Autodesk Fusion 360 part; units mm, degrees
(part 4 of 5)
equation "d84 = FootHeight"
equation "d86 = ( BaseX + LeftRun + FaucetGap ) + ( ( ( RightRun - ModuleGap ) / 2 ) - Wall - 12 mm )"
equation "d87 = ( BaseY ) + ( ( Depth ) - Wall - 12 mm )"
equation "d90 = PanHeight - DeckThick"
equation "d94 = ( BaseX + LeftRun + FaucetGap ) + ( 3 mm )"
equation "d95 = ( BaseY ) + ( 0 mm )"
equation "d96 = RunnerWidth"
equation "d97 = ( Depth ) - 9 mm"
equation "d98 = FootHeight"
equation "d102 = ( BaseX + LeftRun + FaucetGap ) + ( ( ( RightRun - ModuleGap ) / 2 ) - 3 mm - RunnerWidth )"
equation "d103 = ( BaseY ) + ( 0 mm )"
equation "d104 = RunnerWidth"
equation "d105 = ( Depth ) - 9 mm"
equation "d106 = FootHeight"
equation "d108 = TouchChamfer"
equation "d109 = ( FootHeight ) + PanHeight - DeckThick"
equation "d111 = ( BaseX + LeftRun + FaucetGap ) + ( Wall + DeckClearance )"
equation "d112 = ( BaseY ) + ( Wall + DeckClearance )"
equation "d113 = ( ( RightRun - ModuleGap ) / 2 ) - 2 * ( Wall + DeckClearance )"
equation "d114 = ( Depth ) - 2 * ( Wall + DeckClearance )"
equation "d115 = DeckThick"
equation "d117 = ( FootHeight ) + PanHeight - DeckThick"
equation "d119 = ( BaseX + LeftRun + FaucetGap ) + ( ( ( ( ( RightRun - ModuleGap ) / 2 ) - ( 10 * SlotPitch + SlotWidth ) ) / 2 ) + ( 0 * SlotPitch ) )"
equation "d120 = ( BaseY ) + ( Wall + DeckClearance + RimBorder )"
equation "d121 = SlotWidth"
equation "d122 = ( Depth ) - 2 * ( Wall + DeckClearance + RimBorder )"
equation "d123 = DeckThick"
equation "d125 = ( FootHeight ) + PanHeight - DeckThick"
equation "d127 = ( BaseX + LeftRun + FaucetGap ) + ( ( ( ( ( RightRun - ModuleGap ) / 2 ) - ( 10 * SlotPitch + SlotWidth ) ) / 2 ) + ( 1 * SlotPitch ) )"
equation "d128 = ( BaseY ) + ( Wall + DeckClearance + RimBorder )"
equation "d129 = SlotWidth"
equation "d130 = ( Depth ) - 2 * ( Wall + DeckClearance + RimBorder )"
equation "d131 = DeckThick"
equation "d133 = ( FootHeight ) + PanHeight - DeckThick"
equation "d135 = ( BaseX + LeftRun + FaucetGap ) + ( ( ( ( ( RightRun - ModuleGap ) / 2 ) - ( 10 * SlotPitch + SlotWidth ) ) / 2 ) + ( 2 * SlotPitch ) )"
equation "d136 = ( BaseY ) + ( Wall + DeckClearance + RimBorder )"
equation "d137 = SlotWidth"
equation "d138 = ( Depth ) - 2 * ( Wall + DeckClearance + RimBorder )"
equation "d139 = DeckThick"
equation "d141 = ( FootHeight ) + PanHeight - DeckThick"
equation "d143 = ( BaseX + LeftRun + FaucetGap ) + ( ( ( ( ( RightRun - ModuleGap ) / 2 ) - ( 10 * SlotPitch + SlotWidth ) ) / 2 ) + ( 3 * SlotPitch ) )"
equation "d144 = ( BaseY ) + ( Wall + DeckClearance + RimBorder )"
equation "d145 = SlotWidth"
equation "d146 = ( Depth ) - 2 * ( Wall + DeckClearance + RimBorder )"
equation "d147 = DeckThick"
equation "d149 = ( FootHeight ) + PanHeight - DeckThick"
equation "d151 = ( BaseX + LeftRun + FaucetGap ) + ( ( ( ( ( RightRun - ModuleGap ) / 2 ) - ( 10 * SlotPitch + SlotWidth ) ) / 2 ) + ( 4 * SlotPitch ) )"
equation "d152 = ( BaseY ) + ( Wall + DeckClearance + RimBorder )"
equation "d153 = SlotWidth"
equation "d154 = ( Depth ) - 2 * ( Wall + DeckClearance + RimBorder )"
equation "d155 = DeckThick"
equation "d157 = ( FootHeight ) + PanHeight - DeckThick"
equation "d159 = ( BaseX + LeftRun + FaucetGap ) + ( ( ( ( ( RightRun - ModuleGap ) / 2 ) - ( 10 * SlotPitch + SlotWidth ) ) / 2 ) + ( 5 * SlotPitch ) )"
equation "d160 = ( BaseY ) + ( Wall + DeckClearance + RimBorder )"
equation "d161 = SlotWidth"
equation "d162 = ( Depth ) - 2 * ( Wall + DeckClearance + RimBorder )"
equation "d163 = DeckThick"
equation "d165 = ( FootHeight ) + PanHeight - DeckThick"
equation "d167 = ( BaseX + LeftRun + FaucetGap ) + ( ( ( ( ( RightRun - ModuleGap ) / 2 ) - ( 10 * SlotPitch + SlotWidth ) ) / 2 ) + ( 6 * SlotPitch ) )"
equation "d168 = ( BaseY ) + ( Wall + DeckClearance + RimBorder )"
equation "d169 = SlotWidth"
equation "d170 = ( Depth ) - 2 * ( Wall + DeckClearance + RimBorder )"
equation "d171 = DeckThick"
equation "d173 = ( FootHeight ) + PanHeight - DeckThick"
equation "d175 = ( BaseX + LeftRun + FaucetGap ) + ( ( ( ( ( RightRun - ModuleGap ) / 2 ) - ( 10 * SlotPitch + SlotWidth ) ) / 2 ) + ( 7 * SlotPitch ) )"
equation "d176 = ( BaseY ) + ( Wall + DeckClearance + RimBorder )"
equation "d177 = SlotWidth"
equation "d178 = ( Depth ) - 2 * ( Wall + DeckClearance + RimBorder )"
equation "d179 = DeckThick"
equation "d181 = ( FootHeight ) + PanHeight - DeckThick"
equation "d183 = ( BaseX + LeftRun + FaucetGap ) + ( ( ( ( ( RightRun - ModuleGap ) / 2 ) - ( 10 * SlotPitch + SlotWidth ) ) / 2 ) + ( 8 * SlotPitch ) )"
equation "d184 = ( BaseY ) + ( Wall + DeckClearance + RimBorder )"
equation "d185 = SlotWidth"
equation "d186 = ( Depth ) - 2 * ( Wall + DeckClearance + RimBorder )"
equation "d187 = DeckThick"
equation "d189 = ( FootHeight ) + PanHeight - DeckThick"
equation "d191 = ( BaseX + LeftRun + FaucetGap ) + ( ( ( ( ( RightRun - ModuleGap ) / 2 ) - ( 10 * SlotPitch + SlotWidth ) ) / 2 ) + ( 9 * SlotPitch ) )"
equation "d192 = ( BaseY ) + ( Wall + DeckClearance + RimBorder )"
equation "d193 = SlotWidth"
equation "d194 = ( Depth ) - 2 * ( Wall + DeckClearance + RimBorder )"
equation "d195 = DeckThick"
equation "d197 = ( FootHeight ) + PanHeight - DeckThick"
equation "d199 = ( BaseX + LeftRun + FaucetGap ) + ( ( ( ( ( RightRun - ModuleGap ) / 2 ) - ( 10 * SlotPitch + SlotWidth ) ) / 2 ) + ( 10 * SlotPitch ) )"
equation "d200 = ( BaseY ) + ( Wall + DeckClearance + RimBorder )"
equation "d201 = SlotWidth"
equation "d202 = ( Depth ) - 2 * ( Wall + DeckClearance + RimBorder )"
equation "d203 = DeckThick"
equation "d205 = ( FootHeight ) + PanHeight - DeckThick"
equation "d207 = ( BaseX + LeftRun + FaucetGap ) + ( ( ( RightRun - ModuleGap ) / 2 ) / 2 - 8 mm )"
equation "d208 = ( BaseY ) + ( ( Depth ) - Wall - DeckClearance - 4 mm )"
equation "d211 = DeckThick"
equation "d213 = TouchChamfer"
equation "d214 = FootHeight"
equation "d216 = ( BaseX ) + ( 0 mm )"
equation "d217 = ( BaseY ) + ( 0 mm )"
equation "d218 = TowerWidth"
equation "d219 = Depth"
equation "d220 = PanHeight"
equation "d224 = ( BaseX ) + ( Wall )"
equation "d226 = -( -( ( FootHeight ) + FloorMin + ( ( Depth ) - ( Wall ) ) * tan(DrainSlope) ) )"
equation "d227 = ( ( BaseY ) + ( Wall ) )"
equation "d228 = -( -( ( FootHeight ) + FloorMin + ( ( Depth ) - ( Depth ) ) * tan(DrainSlope) ) )"
equation "d229 = ( ( BaseY ) + ( Depth ) )"
equation "d230 = -( -( FootHeight + PanHeight + 1 mm ) )"
equation "d231 = ( TowerWidth ) - 2 * Wall"
equation "d233 = FootHeight"
equation "d235 = ( BaseX ) + ( Wall )"
equation "d236 = ( BaseY ) + ( Wall )"
equation "d239 = PanHeight - DeckThick"
equation "d241 = FootHeight"
equation "d243 = ( BaseX ) + ( Wall )"
equation "d244 = ( BaseY ) + ( ( Depth ) - Wall - 12 mm )"
equation "d247 = PanHeight - DeckThick"
equation "d249 = FootHeight"
equation "d251 = ( BaseX ) + ( ( TowerWidth ) - Wall - 12 mm )"
equation "d252 = ( BaseY ) + ( Wall )"
equation "d255 = PanHeight - DeckThick"
equation "d257 = FootHeight"
equation "d259 = ( BaseX ) + ( ( TowerWidth ) - Wall - 12 mm )"
equation "d260 = ( BaseY ) + ( ( Depth ) - Wall - 12 mm )"
equation "d263 = PanHeight - DeckThick"
equation "d267 = ( BaseX ) + ( 3 mm )"
equation "d268 = ( BaseY ) + ( 0 mm )"
equation "d269 = RunnerWidth"
equation "d270 = ( Depth ) - 9 mm"
equation "d271 = FootHeight"
equation "d275 = ( BaseX ) + ( ( TowerWidth ) - 3 mm - RunnerWidth )"
equation "d276 = ( BaseY ) + ( 0 mm )"
equation "d277 = RunnerWidth"
equation "d278 = ( Depth ) - 9 mm"
equation "d279 = FootHeight"
equation "d281 = TouchChamfer"
equation "d282 = ( FootHeight ) + PanHeight - DeckThick"
equation "d284 = ( BaseX ) + ( Wall + DeckClearance )"
equation "d285 = ( BaseY ) + ( Wall + DeckClearance )"
equation "d286 = ( TowerWidth ) - 2 * ( Wall + DeckClearance )"
equation "d287 = ( Depth ) - 2 * ( Wall + DeckClearance )"
equation "d288 = DeckThick"
equation "d290 = ( FootHeight ) + PanHeight - DeckThick"
equation "d292 = ( BaseX ) + ( ( ( ( TowerWidth ) - ( 14 * SlotPitch + SlotWidth ) ) / 2 ) + ( 0 * SlotPitch ) )"
equation "d293 = ( BaseY ) + ( Wall + DeckClearance + RimBorder )"
equation "d294 = SlotWidth"
equation "d295 = ( Depth ) - 2 * ( Wall + DeckClearance + RimBorder )"
equation "d296 = DeckThick"
equation "d298 = ( FootHeight ) + PanHeight - DeckThick"
equation "d300 = ( BaseX ) + ( ( ( ( TowerWidth ) - ( 14 * SlotPitch + SlotWidth ) ) / 2 ) + ( 1 * SlotPitch ) )"
equation "d301 = ( BaseY ) + ( Wall + DeckClearance + RimBorder )"
equation "d302 = SlotWidth"
equation "d303 = ( Depth ) - 2 * ( Wall + DeckClearance + RimBorder )"
equation "d304 = DeckThick"
equation "d306 = ( FootHeight ) + PanHeight - DeckThick"
equation "d308 = ( BaseX ) + ( ( ( ( TowerWidth ) - ( 14 * SlotPitch + SlotWidth ) ) / 2 ) + ( 2 * SlotPitch ) )"
equation "d309 = ( BaseY ) + ( Wall + DeckClearance + RimBorder )"
equation "d310 = SlotWidth"
equation "d311 = ( Depth ) - 2 * ( Wall + DeckClearance + RimBorder )"
equation "d312 = DeckThick"
equation "d314 = ( FootHeight ) + PanHeight - DeckThick"
equation "d316 = ( BaseX ) + ( ( ( ( TowerWidth ) - ( 14 * SlotPitch + SlotWidth ) ) / 2 ) + ( 3 * SlotPitch ) )"
equation "d317 = ( BaseY ) + ( Wall + DeckClearance + RimBorder )"
equation "d318 = SlotWidth"
equation "d319 = ( Depth ) - 2 * ( Wall + DeckClearance + RimBorder )"
equation "d320 = DeckThick"
equation "d322 = ( FootHeight ) + PanHeight - DeckThick"
equation "d324 = ( BaseX ) + ( ( ( ( TowerWidth ) - ( 14 * SlotPitch + SlotWidth ) ) / 2 ) + ( 4 * SlotPitch ) )"
equation "d325 = ( BaseY ) + ( Wall + DeckClearance + RimBorder )"
equation "d326 = SlotWidth"
equation "d327 = ( Depth ) - 2 * ( Wall + DeckClearance + RimBorder )"
equation "d328 = DeckThick"
equation "d330 = ( FootHeight ) + PanHeight - DeckThick"
equation "d332 = ( BaseX ) + ( ( ( ( TowerWidth ) - ( 14 * SlotPitch + SlotWidth ) ) / 2 ) + ( 5 * SlotPitch ) )"
equation "d333 = ( BaseY ) + ( Wall + DeckClearance + RimBorder )"
equation "d334 = SlotWidth"
equation "d335 = ( Depth ) - 2 * ( Wall + DeckClearance + RimBorder )"
equation "d336 = DeckThick"
equation "d338 = ( FootHeight ) + PanHeight - DeckThick"
equation "d340 = ( BaseX ) + ( ( ( ( TowerWidth ) - ( 14 * SlotPitch + SlotWidth ) ) / 2 ) + ( 6 * SlotPitch ) )"
equation "d341 = ( BaseY ) + ( Wall + DeckClearance + RimBorder )"
equation "d342 = SlotWidth"
equation "d343 = ( Depth ) - 2 * ( Wall + DeckClearance + RimBorder )"
equation "d344 = DeckThick"
equation "d346 = ( FootHeight ) + PanHeight - DeckThick"
equation "d348 = ( BaseX ) + ( ( ( ( TowerWidth ) - ( 14 * SlotPitch + SlotWidth ) ) / 2 ) + ( 7 * SlotPitch ) )"
equation "d349 = ( BaseY ) + ( Wall + DeckClearance + RimBorder )"
equation "d350 = SlotWidth"
equation "d351 = ( Depth ) - 2 * ( Wall + DeckClearance + RimBorder )"
equation "d352 = DeckThick"
equation "d354 = ( FootHeight ) + PanHeight - DeckThick"
equation "d356 = ( BaseX ) + ( ( ( ( TowerWidth ) - ( 14 * SlotPitch + SlotWidth ) ) / 2 ) + ( 8 * SlotPitch ) )"
equation "d357 = ( BaseY ) + ( Wall + DeckClearance + RimBorder )"
equation "d358 = SlotWidth"
equation "d359 = ( Depth ) - 2 * ( Wall + DeckClearance + RimBorder )"
equation "d360 = DeckThick"
equation "d362 = ( FootHeight ) + PanHeight - DeckThick"
equation "d364 = ( BaseX ) + ( ( ( ( TowerWidth ) - ( 14 * SlotPitch + SlotWidth ) ) / 2 ) + ( 9 * SlotPitch ) )"
equation "d365 = ( BaseY ) + ( Wall + DeckClearance + RimBorder )"
equation "d366 = SlotWidth"
equation "d367 = ( Depth ) - 2 * ( Wall + DeckClearance + RimBorder )"
equation "d368 = DeckThick"
equation "d370 = ( FootHeight ) + PanHeight - DeckThick"
equation "d372 = ( BaseX ) + ( ( ( ( TowerWidth ) - ( 14 * SlotPitch + SlotWidth ) ) / 2 ) + ( 10 * SlotPitch ) )"
equation "d373 = ( BaseY ) + ( Wall + DeckClearance + RimBorder )"
equation "d374 = SlotWidth"
equation "d375 = ( Depth ) - 2 * ( Wall + DeckClearance + RimBorder )"
equation "d376 = DeckThick"
equation "d378 = ( FootHeight ) + PanHeight - DeckThick"
equation "d380 = ( BaseX ) + ( ( ( ( TowerWidth ) - ( 14 * SlotPitch + SlotWidth ) ) / 2 ) + ( 11 * SlotPitch ) )"
equation "d381 = ( BaseY ) + ( Wall + DeckClearance + RimBorder )"
equation "d382 = SlotWidth"
equation "d383 = ( Depth ) - 2 * ( Wall + DeckClearance + RimBorder )"
equation "d384 = DeckThick"
equation "d386 = ( FootHeight ) + PanHeight - DeckThick"
equation "d388 = ( BaseX ) + ( ( ( ( TowerWidth ) - ( 14 * SlotPitch + SlotWidth ) ) / 2 ) + ( 12 * SlotPitch ) )"
equation "d389 = ( BaseY ) + ( Wall + DeckClearance + RimBorder )"
equation "d390 = SlotWidth"
equation "d391 = ( Depth ) - 2 * ( Wall + DeckClearance + RimBorder )"
equation "d392 = DeckThick"
equation "d394 = ( FootHeight ) + PanHeight - DeckThick"
equation "d396 = ( BaseX ) + ( ( ( ( TowerWidth ) - ( 14 * SlotPitch + SlotWidth ) ) / 2 ) + ( 13 * SlotPitch ) )"
equation "d397 = ( BaseY ) + ( Wall + DeckClearance + RimBorder )"
equation "d398 = SlotWidth"
equation "d399 = ( Depth ) - 2 * ( Wall + DeckClearance + RimBorder )"
equation "d400 = DeckThick"
equation "d402 = ( FootHeight ) + PanHeight - DeckThick"
equation "d404 = ( BaseX ) + ( ( ( ( TowerWidth ) - ( 14 * SlotPitch + SlotWidth ) ) / 2 ) + ( 14 * SlotPitch ) )"
equation "d405 = ( BaseY ) + ( Wall + DeckClearance + RimBorder )"
equation "d406 = SlotWidth"
equation "d407 = ( Depth ) - 2 * ( Wall + DeckClearance + RimBorder )"
equation "d408 = DeckThick"
equation "d410 = ( FootHeight ) + PanHeight - DeckThick"
equation "d412 = ( BaseX ) + ( ( TowerWidth ) / 2 - 8 mm )"
equation "d413 = ( BaseY ) + ( ( Depth ) - Wall - DeckClearance - 4 mm )"
equation "d416 = DeckThick"
equation "d418 = TouchChamfer"
equation "d419 = FootHeight"
equation "d421 = ( BaseX + TowerWidth + ModuleGap ) + ( 0 mm )"
equation "d422 = ( BaseY ) + ( 0 mm )"
equation "d423 = LeftRun - TowerWidth - ModuleGap"
equation "d424 = Depth"
equation "d425 = PanHeight"
equation "d429 = ( BaseX + TowerWidth + ModuleGap ) + ( Wall )"
equation "d431 = -( -( ( FootHeight ) + FloorMin + ( ( Depth ) - ( Wall ) ) * tan(DrainSlope) ) )"
equation "d432 = ( ( BaseY ) + ( Wall ) )"
equation "d433 = -( -( ( FootHeight ) + FloorMin + ( ( Depth ) - ( Depth ) ) * tan(DrainSlope) ) )"
equation "d434 = ( ( BaseY ) + ( Depth ) )"
equation "d435 = -( -( FootHeight + PanHeight + 1 mm ) )"
equation "d436 = ( LeftRun - TowerWidth - ModuleGap ) - 2 * Wall"
equation "d438 = FootHeight"
equation "d440 = ( BaseX + TowerWidth + ModuleGap ) + ( Wall )"
equation "d441 = ( BaseY ) + ( Wall )"
equation "d444 = PanHeight - DeckThick"
equation "d446 = FootHeight"
equation "d448 = ( BaseX + TowerWidth + ModuleGap ) + ( Wall )"
equation "d449 = ( BaseY ) + ( ( Depth ) - Wall - 12 mm )"
equation "d452 = PanHeight - DeckThick"
equation "d454 = FootHeight"
equation "d456 = ( BaseX + TowerWidth + ModuleGap ) + ( ( LeftRun - TowerWidth - ModuleGap ) - Wall - 12 mm )"
equation "d457 = ( BaseY ) + ( Wall )"
equation "d460 = PanHeight - DeckThick"
equation "d462 = FootHeight"
equation "d464 = ( BaseX + TowerWidth + ModuleGap ) + ( ( LeftRun - TowerWidth - ModuleGap ) - Wall - 12 mm )"
equation "d465 = ( BaseY ) + ( ( Depth ) - Wall - 12 mm )"
equation "d468 = PanHeight - DeckThick"
equation "d472 = ( BaseX + TowerWidth + ModuleGap ) + ( 3 mm )"
equation "d473 = ( BaseY ) + ( 0 mm )"
equation "d474 = RunnerWidth"
equation "d475 = ( Depth ) - 9 mm"
equation "d476 = FootHeight"
equation "d480 = ( BaseX + TowerWidth + ModuleGap ) + ( ( LeftRun - TowerWidth - ModuleGap ) - 3 mm - RunnerWidth )"
equation "d481 = ( BaseY ) + ( 0 mm )"
equation "d482 = RunnerWidth"
equation "d483 = ( Depth ) - 9 mm"
equation "d484 = FootHeight"
equation "d486 = TouchChamfer"
equation "d487 = ( FootHeight ) + PanHeight - DeckThick"
equation "d489 = ( BaseX + TowerWidth + ModuleGap ) + ( Wall + DeckClearance )"
equation "d490 = ( BaseY ) + ( Wall + DeckClearance )"
equation "d491 = ( LeftRun - TowerWidth - ModuleGap ) - 2 * ( Wall + DeckClearance )"
equation "d492 = ( Depth ) - 2 * ( Wall + DeckClearance )"
equation "d493 = DeckThick"
equation "d495 = ( FootHeight ) + PanHeight - DeckThick"
equation "d497 = ( BaseX + TowerWidth + ModuleGap ) + ( ( ( ( LeftRun - TowerWidth - ModuleGap ) - ( 16 * SlotPitch + SlotWidth ) ) / 2 ) + ( 0 * SlotPitch ) )"
equation "d498 = ( BaseY ) + ( Wall + DeckClearance + RimBorder )"
equation "d499 = SlotWidth"
equation "d500 = ( Depth ) - 2 * ( Wall + DeckClearance + RimBorder )"
equation "d501 = DeckThick"
equation "d503 = ( FootHeight ) + PanHeight - DeckThick"
equation "d505 = ( BaseX + TowerWidth + ModuleGap ) + ( ( ( ( LeftRun - TowerWidth - ModuleGap ) - ( 16 * SlotPitch + SlotWidth ) ) / 2 ) + ( 1 * SlotPitch ) )"
equation "d506 = ( BaseY ) + ( Wall + DeckClearance + RimBorder )"
equation "d507 = SlotWidth"
equation "d508 = ( Depth ) - 2 * ( Wall + DeckClearance + RimBorder )"
equation "d509 = DeckThick"
equation "d511 = ( FootHeight ) + PanHeight - DeckThick"
equation "d513 = ( BaseX + TowerWidth + ModuleGap ) + ( ( ( ( LeftRun - TowerWidth - ModuleGap ) - ( 16 * SlotPitch + SlotWidth ) ) / 2 ) + ( 2 * SlotPitch ) )"
equation "d514 = ( BaseY ) + ( Wall + DeckClearance + RimBorder )"
equation "d515 = SlotWidth"
equation "d516 = ( Depth ) - 2 * ( Wall + DeckClearance + RimBorder )"
equation "d517 = DeckThick"
equation "d519 = ( FootHeight ) + PanHeight - DeckThick"
equation "d521 = ( BaseX + TowerWidth + ModuleGap ) + ( ( ( ( LeftRun - TowerWidth - ModuleGap ) - ( 16 * SlotPitch + SlotWidth ) ) / 2 ) + ( 3 * SlotPitch ) )"
equation "d522 = ( BaseY ) + ( Wall + DeckClearance + RimBorder )"
equation "d523 = SlotWidth"
equation "d524 = ( Depth ) - 2 * ( Wall + DeckClearance + RimBorder )"
equation "d525 = DeckThick"
equation "d527 = ( FootHeight ) + PanHeight - DeckThick"
equation "d529 = ( BaseX + TowerWidth + ModuleGap ) + ( ( ( ( LeftRun - TowerWidth - ModuleGap ) - ( 16 * SlotPitch + SlotWidth ) ) / 2 ) + ( 4 * SlotPitch ) )"
equation "d530 = ( BaseY ) + ( Wall + DeckClearance + RimBorder )"
equation "d531 = SlotWidth"
equation "d532 = ( Depth ) - 2 * ( Wall + DeckClearance + RimBorder )"
equation "d533 = DeckThick"
equation "d535 = ( FootHeight ) + PanHeight - DeckThick"
equation "d537 = ( BaseX + TowerWidth + ModuleGap ) + ( ( ( ( LeftRun - TowerWidth - ModuleGap ) - ( 16 * SlotPitch + SlotWidth ) ) / 2 ) + ( 5 * SlotPitch ) )"
equation "d538 = ( BaseY ) + ( Wall + DeckClearance + RimBorder )"
equation "d539 = SlotWidth"
equation "d540 = ( Depth ) - 2 * ( Wall + DeckClearance + RimBorder )"
equation "d541 = DeckThick"
equation "d543 = ( FootHeight ) + PanHeight - DeckThick"
equation "d545 = ( BaseX + TowerWidth + ModuleGap ) + ( ( ( ( LeftRun - TowerWidth - ModuleGap ) - ( 16 * SlotPitch + SlotWidth ) ) / 2 ) + ( 6 * SlotPitch ) )"
equation "d546 = ( BaseY ) + ( Wall + DeckClearance + RimBorder )"
equation "d547 = SlotWidth"
equation "d548 = ( Depth ) - 2 * ( Wall + DeckClearance + RimBorder )"
equation "d549 = DeckThick"
equation "d551 = ( FootHeight ) + PanHeight - DeckThick"
equation "d553 = ( BaseX + TowerWidth + ModuleGap ) + ( ( ( ( LeftRun - TowerWidth - ModuleGap ) - ( 16 * SlotPitch + SlotWidth ) ) / 2 ) + ( 7 * SlotPitch ) )"
equation "d554 = ( BaseY ) + ( Wall + DeckClearance + RimBorder )"
equation "d555 = SlotWidth"
equation "d556 = ( Depth ) - 2 * ( Wall + DeckClearance + RimBorder )"
equation "d557 = DeckThick"
equation "d559 = ( FootHeight ) + PanHeight - DeckThick"
equation "d561 = ( BaseX + TowerWidth + ModuleGap ) + ( ( ( ( LeftRun - TowerWidth - ModuleGap ) - ( 16 * SlotPitch + SlotWidth ) ) / 2 ) + ( 8 * SlotPitch ) )"
equation "d562 = ( BaseY ) + ( Wall + DeckClearance + RimBorder )"
equation "d563 = SlotWidth"
equation "d564 = ( Depth ) - 2 * ( Wall + DeckClearance + RimBorder )"
equation "d565 = DeckThick"
equation "d567 = ( FootHeight ) + PanHeight - DeckThick"
equation "d569 = ( BaseX + TowerWidth + ModuleGap ) + ( ( ( ( LeftRun - TowerWidth - ModuleGap ) - ( 16 * SlotPitch + SlotWidth ) ) / 2 ) + ( 9 * SlotPitch ) )"
equation "d570 = ( BaseY ) + ( Wall + DeckClearance + RimBorder )"
equation "d571 = SlotWidth"
equation "d572 = ( Depth ) - 2 * ( Wall + DeckClearance + RimBorder )"
equation "d573 = DeckThick"
equation "d575 = ( FootHeight ) + PanHeight - DeckThick"
equation "d577 = ( BaseX + TowerWidth + ModuleGap ) + ( ( ( ( LeftRun - TowerWidth - ModuleGap ) - ( 16 * SlotPitch + SlotWidth ) ) / 2 ) + ( 10 * SlotPitch ) )"
equation "d578 = ( BaseY ) + ( Wall + DeckClearance + RimBorder )"
equation "d579 = SlotWidth"
equation "d580 = ( Depth ) - 2 * ( Wall + DeckClearance + RimBorder )"
equation "d581 = DeckThick"
equation "d583 = ( FootHeight ) + PanHeight - DeckThick"
equation "d585 = ( BaseX + TowerWidth + ModuleGap ) + ( ( ( ( LeftRun - TowerWidth - ModuleGap ) - ( 16 * SlotPitch + SlotWidth ) ) / 2 ) + ( 11 * SlotPitch ) )"
equation "d586 = ( BaseY ) + ( Wall + DeckClearance + RimBorder )"
equation "d587 = SlotWidth"
equation "d588 = ( Depth ) - 2 * ( Wall + DeckClearance + RimBorder )"
equation "d589 = DeckThick"
equation "d591 = ( FootHeight ) + PanHeight - DeckThick"
equation "d593 = ( BaseX + TowerWidth + ModuleGap ) + ( ( ( ( LeftRun - TowerWidth - ModuleGap ) - ( 16 * SlotPitch + SlotWidth ) ) / 2 ) + ( 12 * SlotPitch ) )"
equation "d594 = ( BaseY ) + ( Wall + DeckClearance + RimBorder )"
equation "d595 = SlotWidth"
equation "d596 = ( Depth ) - 2 * ( Wall + DeckClearance + RimBorder )"
equation "d597 = DeckThick"
equation "d599 = ( FootHeight ) + PanHeight - DeckThick"
equation "d601 = ( BaseX + TowerWidth + ModuleGap ) + ( ( ( ( LeftRun - TowerWidth - ModuleGap ) - ( 16 * SlotPitch + SlotWidth ) ) / 2 ) + ( 13 * SlotPitch ) )"
equation "d602 = ( BaseY ) + ( Wall + DeckClearance + RimBorder )"
equation "d603 = SlotWidth"
equation "d604 = ( Depth ) - 2 * ( Wall + DeckClearance + RimBorder )"
equation "d605 = DeckThick"
equation "d607 = ( FootHeight ) + PanHeight - DeckThick"
equation "d609 = ( BaseX + TowerWidth + ModuleGap ) + ( ( ( ( LeftRun - TowerWidth - ModuleGap ) - ( 16 * SlotPitch + SlotWidth ) ) / 2 ) + ( 14 * SlotPitch ) )"
equation "d610 = ( BaseY ) + ( Wall + DeckClearance + RimBorder )"
equation "d611 = SlotWidth"
equation "d612 = ( Depth ) - 2 * ( Wall + DeckClearance + RimBorder )"
equation "d613 = DeckThick"
equation "d615 = ( FootHeight ) + PanHeight - DeckThick"
equation "d617 = ( BaseX + TowerWidth + ModuleGap ) + ( ( ( ( LeftRun - TowerWidth - ModuleGap ) - ( 16 * SlotPitch + SlotWidth ) ) / 2 ) + ( 15 * SlotPitch ) )"
equation "d618 = ( BaseY ) + ( Wall + DeckClearance + RimBorder )"
equation "d619 = SlotWidth"
equation "d620 = ( Depth ) - 2 * ( Wall + DeckClearance + RimBorder )"
equation "d621 = DeckThick"
equation "d623 = ( FootHeight ) + PanHeight - DeckThick"
equation "d625 = ( BaseX + TowerWidth + ModuleGap ) + ( ( ( ( LeftRun - TowerWidth - ModuleGap ) - ( 16 * SlotPitch + SlotWidth ) ) / 2 ) + ( 16 * SlotPitch ) )"
equation "d626 = ( BaseY ) + ( Wall + DeckClearance + RimBorder )"
equation "d627 = SlotWidth"
equation "d628 = ( Depth ) - 2 * ( Wall + DeckClearance + RimBorder )"
equation "d629 = DeckThick"
equation "d631 = ( FootHeight ) + PanHeight - DeckThick"
equation "d633 = ( BaseX + TowerWidth + ModuleGap ) + ( ( LeftRun - TowerWidth - ModuleGap ) / 2 - 8 mm )"
equation "d634 = ( BaseY ) + ( ( Depth ) - Wall - DeckClearance - 4 mm )"
equation "d637 = DeckThick"
equation "d639 = TouchChamfer"
equation "d640 = FootHeight"
equation "d642 = ( BaseX + LeftRun + FaucetGap + ( RightRun + ModuleGap ) / 2 ) + ( 0 mm )"
equation "d643 = ( BaseY ) + ( 0 mm )"
equation "d644 = ( RightRun - ModuleGap ) / 2"
equation "d645 = Depth"
equation "d646 = PanHeight"
equation "d650 = ( BaseX + LeftRun + FaucetGap + ( RightRun + ModuleGap ) / 2 ) + ( Wall )"
equation "d652 = -( -( ( FootHeight ) + FloorMin + ( ( Depth ) - ( Wall ) ) * tan(DrainSlope) ) )"
equation "d653 = ( ( BaseY ) + ( Wall ) )"
equation "d654 = -( -( ( FootHeight ) + FloorMin + ( ( Depth ) - ( Depth ) ) * tan(DrainSlope) ) )"
equation "d655 = ( ( BaseY ) + ( Depth ) )"
equation "d656 = -( -( FootHeight + PanHeight + 1 mm ) )"
equation "d657 = ( ( RightRun - ModuleGap ) / 2 ) - 2 * Wall"
equation "d659 = FootHeight"
equation "d661 = ( BaseX + LeftRun + FaucetGap + ( RightRun + ModuleGap ) / 2 ) + ( Wall )"
equation "d662 = ( BaseY ) + ( Wall )"
equation "d665 = PanHeight - DeckThick"
equation "d667 = FootHeight"
equation "d669 = ( BaseX + LeftRun + FaucetGap + ( RightRun + ModuleGap ) / 2 ) + ( Wall )"
equation "d670 = ( BaseY ) + ( ( Depth ) - Wall - 12 mm )"
equation "d673 = PanHeight - DeckThick"
equation "d675 = FootHeight"
equation "d677 = ( BaseX + LeftRun + FaucetGap + ( RightRun + ModuleGap ) / 2 ) + ( ( ( RightRun - ModuleGap ) / 2 ) - Wall - 12 mm )"
equation "d678 = ( BaseY ) + ( Wall )"
equation "d681 = PanHeight - DeckThick"
equation "d683 = FootHeight"
equation "d685 = ( BaseX + LeftRun + FaucetGap + ( RightRun + ModuleGap ) / 2 ) + ( ( ( RightRun - ModuleGap ) / 2 ) - Wall - 12 mm )"
equation "d686 = ( BaseY ) + ( ( Depth ) - Wall - 12 mm )"
equation "d689 = PanHeight - DeckThick"
equation "d693 = ( BaseX + LeftRun + FaucetGap + ( RightRun + ModuleGap ) / 2 ) + ( 3 mm )"
equation "d694 = ( BaseY ) + ( 0 mm )"
equation "d695 = RunnerWidth"
equation "d696 = ( Depth ) - 9 mm"
equation "d697 = FootHeight"
equation "d701 = ( BaseX + LeftRun + FaucetGap + ( RightRun + ModuleGap ) / 2 ) + ( ( ( RightRun - ModuleGap ) / 2 ) - 3 mm - RunnerWidth )"
equation "d702 = ( BaseY ) + ( 0 mm )"
equation "d703 = RunnerWidth"
equation "d704 = ( Depth ) - 9 mm"
equation "d705 = FootHeight"
equation "d707 = TouchChamfer"
equation "d708 = ( FootHeight ) + PanHeight - DeckThick"
equation "d710 = ( BaseX + LeftRun + FaucetGap + ( RightRun + ModuleGap ) / 2 ) + ( Wall + DeckClearance )"
equation "d711 = ( BaseY ) + ( Wall + DeckClearance )"
equation "d712 = ( ( RightRun - ModuleGap ) / 2 ) - 2 * ( Wall + DeckClearance )"
equation "d713 = ( Depth ) - 2 * ( Wall + DeckClearance )"
equation "d714 = DeckThick"
equation "d716 = ( FootHeight ) + PanHeight - DeckThick"
equation "d718 = ( BaseX + LeftRun + FaucetGap + ( RightRun + ModuleGap ) / 2 ) + ( ( ( ( ( RightRun - ModuleGap ) / 2 ) - ( 10 * SlotPitch + SlotWidth ) ) / 2 ) + ( 0 * SlotPitch ) )"
equation "d719 = ( BaseY ) + ( Wall + DeckClearance + RimBorder )"
equation "d720 = SlotWidth"
equation "d721 = ( Depth ) - 2 * ( Wall + DeckClearance + RimBorder )"
equation "d722 = DeckThick"
equation "d724 = ( FootHeight ) + PanHeight - DeckThick"
equation "d726 = ( BaseX + LeftRun + FaucetGap + ( RightRun + ModuleGap ) / 2 ) + ( ( ( ( ( RightRun - ModuleGap ) / 2 ) - ( 10 * SlotPitch + SlotWidth ) ) / 2 ) + ( 1 * SlotPitch ) )"
equation "d727 = ( BaseY ) + ( Wall + DeckClearance + RimBorder )"
equation "d728 = SlotWidth"
equation "d729 = ( Depth ) - 2 * ( Wall + DeckClearance + RimBorder )"
equation "d730 = DeckThick"
equation "d732 = ( FootHeight ) + PanHeight - DeckThick"
equation "d734 = ( BaseX + LeftRun + FaucetGap + ( RightRun + ModuleGap ) / 2 ) + ( ( ( ( ( RightRun - ModuleGap ) / 2 ) - ( 10 * SlotPitch + SlotWidth ) ) / 2 ) + ( 2 * SlotPitch ) )"
equation "d735 = ( BaseY ) + ( Wall + DeckClearance + RimBorder )"
equation "d736 = SlotWidth"
equation "d737 = ( Depth ) - 2 * ( Wall + DeckClearance + RimBorder )"
equation "d738 = DeckThick"
equation "d740 = ( FootHeight ) + PanHeight - DeckThick"
equation "d742 = ( BaseX + LeftRun + FaucetGap + ( RightRun + ModuleGap ) / 2 ) + ( ( ( ( ( RightRun - ModuleGap ) / 2 ) - ( 10 * SlotPitch + SlotWidth ) ) / 2 ) + ( 3 * SlotPitch ) )"
equation "d743 = ( BaseY ) + ( Wall + DeckClearance + RimBorder )"
equation "d744 = SlotWidth"
equation "d745 = ( Depth ) - 2 * ( Wall + DeckClearance + RimBorder )"
equation "d746 = DeckThick"
equation "d748 = ( FootHeight ) + PanHeight - DeckThick"
equation "d750 = ( BaseX + LeftRun + FaucetGap + ( RightRun + ModuleGap ) / 2 ) + ( ( ( ( ( RightRun - ModuleGap ) / 2 ) - ( 10 * SlotPitch + SlotWidth ) ) / 2 ) + ( 4 * SlotPitch ) )"
equation "d751 = ( BaseY ) + ( Wall + DeckClearance + RimBorder )"
equation "d752 = SlotWidth"
equation "d753 = ( Depth ) - 2 * ( Wall + DeckClearance + RimBorder )"
equation "d754 = DeckThick"
equation "d756 = ( FootHeight ) + PanHeight - DeckThick"
equation "d758 = ( BaseX + LeftRun + FaucetGap + ( RightRun + ModuleGap ) / 2 ) + ( ( ( ( ( RightRun - ModuleGap ) / 2 ) - ( 10 * SlotPitch + SlotWidth ) ) / 2 ) + ( 5 * SlotPitch ) )"
equation "d759 = ( BaseY ) + ( Wall + DeckClearance + RimBorder )"
equation "d760 = SlotWidth"
equation "d761 = ( Depth ) - 2 * ( Wall + DeckClearance + RimBorder )"
equation "d762 = DeckThick"
equation "d764 = ( FootHeight ) + PanHeight - DeckThick"
equation "d766 = ( BaseX + LeftRun + FaucetGap + ( RightRun + ModuleGap ) / 2 ) + ( ( ( ( ( RightRun - ModuleGap ) / 2 ) - ( 10 * SlotPitch + SlotWidth ) ) / 2 ) + ( 6 * SlotPitch ) )"
equation "d767 = ( BaseY ) + ( Wall + DeckClearance + RimBorder )"
equation "d768 = SlotWidth"
equation "d769 = ( Depth ) - 2 * ( Wall + DeckClearance + RimBorder )"
equation "d770 = DeckThick"
equation "d772 = ( FootHeight ) + PanHeight - DeckThick"
equation "d774 = ( BaseX + LeftRun + FaucetGap + ( RightRun + ModuleGap ) / 2 ) + ( ( ( ( ( RightRun - ModuleGap ) / 2 ) - ( 10 * SlotPitch + SlotWidth ) ) / 2 ) + ( 7 * SlotPitch ) )"
equation "d775 = ( BaseY ) + ( Wall + DeckClearance + RimBorder )"
equation "d776 = SlotWidth"
equation "d777 = ( Depth ) - 2 * ( Wall + DeckClearance + RimBorder )"
equation "d778 = DeckThick"
equation "d780 = ( FootHeight ) + PanHeight - DeckThick"
equation "d782 = ( BaseX + LeftRun + FaucetGap + ( RightRun + ModuleGap ) / 2 ) + ( ( ( ( ( RightRun - ModuleGap ) / 2 ) - ( 10 * SlotPitch + SlotWidth ) ) / 2 ) + ( 8 * SlotPitch ) )"
equation "d783 = ( BaseY ) + ( Wall + DeckClearance + RimBorder )"
equation "d784 = SlotWidth"
equation "d785 = ( Depth ) - 2 * ( Wall + DeckClearance + RimBorder )"
equation "d786 = DeckThick"
equation "d788 = ( FootHeight ) + PanHeight - DeckThick"
equation "d790 = ( BaseX + LeftRun + FaucetGap + ( RightRun + ModuleGap ) / 2 ) + ( ( ( ( ( RightRun - ModuleGap ) / 2 ) - ( 10 * SlotPitch + SlotWidth ) ) / 2 ) + ( 9 * SlotPitch ) )"
equation "d791 = ( BaseY ) + ( Wall + DeckClearance + RimBorder )"
equation "d792 = SlotWidth"
equation "d793 = ( Depth ) - 2 * ( Wall + DeckClearance + RimBorder )"
equation "d794 = DeckThick"
equation "d796 = ( FootHeight ) + PanHeight - DeckThick"
equation "d798 = ( BaseX + LeftRun + FaucetGap + ( RightRun + ModuleGap ) / 2 ) + ( ( ( ( ( RightRun - ModuleGap ) / 2 ) - ( 10 * SlotPitch + SlotWidth ) ) / 2 ) + ( 10 * SlotPitch ) )"
equation "d799 = ( BaseY ) + ( Wall + DeckClearance + RimBorder )"
equation "d800 = SlotWidth"
equation "d801 = ( Depth ) - 2 * ( Wall + DeckClearance + RimBorder )"
equation "d802 = DeckThick"
equation "d804 = ( FootHeight ) + PanHeight - DeckThick"
equation "d806 = ( BaseX + LeftRun + FaucetGap + ( RightRun + ModuleGap ) / 2 ) + ( ( ( RightRun - ModuleGap ) / 2 ) / 2 - 8 mm )"
equation "d807 = ( BaseY ) + ( ( Depth ) - Wall - DeckClearance - 4 mm )"
equation "d810 = DeckThick"
equation "d812 = TouchChamfer"
equation "d813 = FootHeight"
equation "d815 = ( BaseX ) + ( 0 mm )"
equation "d816 = ( BaseY + Depth + ModuleGap ) + ( ( LeftReach ) - ( ( 0 mm ) + ( LeftReach ) ) )"
equation "d817 = LeftSideDepth"
equation "d818 = LeftReach"
equation "d819 = PanHeight"
equation "d823 = ( BaseY + Depth + ModuleGap ) + ( ( LeftReach ) - ( Wall ) )"
equation "d825 = ( ( BaseX ) + ( Wall ) )"
equation "d826 = -( -( ( FootHeight ) + FloorMin + ( ( LeftSideDepth ) - ( Wall ) ) * tan(DrainSlope) ) )"
equation "d827 = ( ( BaseX ) + ( LeftSideDepth ) )"
equation "d828 = -( -( ( FootHeight ) + FloorMin + ( ( LeftSideDepth ) - ( LeftSideDepth ) ) * tan(DrainSlope) ) )"
equation "d829 = -( -( FootHeight + PanHeight + 1 mm ) )"
equation "d830 = -( -( -( ( LeftReach ) - 2 * Wall ) ) )"
equation "d832 = FootHeight"
equation "d834 = ( BaseX ) + ( Wall )"
equation "d835 = ( BaseY + Depth + ModuleGap ) + ( ( LeftReach ) - ( ( Wall ) + ( 12 mm ) ) )"
equation "d838 = PanHeight - DeckThick"
equation "d840 = FootHeight"
equation "d842 = ( BaseX ) + ( ( LeftSideDepth ) - Wall - 12 mm )"
equation "d843 = ( BaseY + Depth + ModuleGap ) + ( ( LeftReach ) - ( ( Wall ) + ( 12 mm ) ) )"
equation "d846 = PanHeight - DeckThick"
equation "d848 = FootHeight"
equation "d850 = ( BaseX ) + ( Wall )"
equation "d851 = ( BaseY + Depth + ModuleGap ) + ( ( LeftReach ) - ( ( ( LeftReach ) - Wall - 12 mm ) + ( 12 mm ) ) )"
equation "d854 = PanHeight - DeckThick"
equation "d856 = FootHeight"
equation "d858 = ( BaseX ) + ( ( LeftSideDepth ) - Wall - 12 mm )"
equation "d859 = ( BaseY + Depth + ModuleGap ) + ( ( LeftReach ) - ( ( ( LeftReach ) - Wall - 12 mm ) + ( 12 mm ) ) )"
equation "d862 = PanHeight - DeckThick"
equation "d866 = ( BaseX ) + ( 0 mm )"
equation "d867 = ( BaseY + Depth + ModuleGap ) + ( ( LeftReach ) - ( ( 3 mm ) + ( RunnerWidth ) ) )"
equation "d868 = ( LeftSideDepth ) - 9 mm"
equation "d869 = RunnerWidth"
equation "d870 = FootHeight"
equation "d874 = ( BaseX ) + ( 0 mm )"
equation "d875 = ( BaseY + Depth + ModuleGap ) + ( ( LeftReach ) - ( ( ( LeftReach ) - 3 mm - RunnerWidth ) + ( RunnerWidth ) ) )"
equation "d876 = ( LeftSideDepth ) - 9 mm"
equation "d877 = RunnerWidth"
equation "d878 = FootHeight"
equation "d880 = TouchChamfer"
equation "d881 = ( FootHeight ) + PanHeight - DeckThick"
equation "d883 = ( BaseX ) + ( Wall + DeckClearance )"
equation "d884 = ( BaseY + Depth + ModuleGap ) + ( ( LeftReach ) - ( ( Wall + DeckClearance ) + ( ( LeftReach ) - 2 * ( Wall + DeckClearance ) ) ) )"
equation "d885 = ( LeftSideDepth ) - 2 * ( Wall + DeckClearance )"
equation "d886 = ( LeftReach ) - 2 * ( Wall + DeckClearance )"
equation "d887 = DeckThick"
equation "d889 = ( FootHeight ) + PanHeight - DeckThick"
equation "d891 = ( BaseX ) + ( Wall + DeckClearance + RimBorder )"
equation "d892 = ( BaseY + Depth + ModuleGap ) + ( ( LeftReach ) - ( ( ( ( ( LeftReach ) - ( 14 * SlotPitch + SlotWidth ) ) / 2 ) + ( 0 * SlotPitch ) ) + ( SlotWidth ) ) )"
equation "d893 = ( LeftSideDepth ) - 2 * ( Wall + DeckClearance + RimBorder )"
equation "d894 = SlotWidth"
equation "d895 = DeckThick"
equation "d897 = ( FootHeight ) + PanHeight - DeckThick"
equation "d899 = ( BaseX ) + ( Wall + DeckClearance + RimBorder )"
equation "d900 = ( BaseY + Depth + ModuleGap ) + ( ( LeftReach ) - ( ( ( ( ( LeftReach ) - ( 14 * SlotPitch + SlotWidth ) ) / 2 ) + ( 1 * SlotPitch ) ) + ( SlotWidth ) ) )"
equation "d901 = ( LeftSideDepth ) - 2 * ( Wall + DeckClearance + RimBorder )"
equation "d902 = SlotWidth"
equation "d903 = DeckThick"
equation "d905 = ( FootHeight ) + PanHeight - DeckThick"
equation "d907 = ( BaseX ) + ( Wall + DeckClearance + RimBorder )"
equation "d908 = ( BaseY + Depth + ModuleGap ) + ( ( LeftReach ) - ( ( ( ( ( LeftReach ) - ( 14 * SlotPitch + SlotWidth ) ) / 2 ) + ( 2 * SlotPitch ) ) + ( SlotWidth ) ) )"
equation "d909 = ( LeftSideDepth ) - 2 * ( Wall + DeckClearance + RimBorder )"
equation "d910 = SlotWidth"
equation "d911 = DeckThick"
equation "d913 = ( FootHeight ) + PanHeight - DeckThick"
equation "d915 = ( BaseX ) + ( Wall + DeckClearance + RimBorder )"
equation "d916 = ( BaseY + Depth + ModuleGap ) + ( ( LeftReach ) - ( ( ( ( ( LeftReach ) - ( 14 * SlotPitch + SlotWidth ) ) / 2 ) + ( 3 * SlotPitch ) ) + ( SlotWidth ) ) )"
equation "d917 = ( LeftSideDepth ) - 2 * ( Wall + DeckClearance + RimBorder )"
equation "d918 = SlotWidth"
equation "d919 = DeckThick"
equation "d921 = ( FootHeight ) + PanHeight - DeckThick"
equation "d923 = ( BaseX ) + ( Wall + DeckClearance + RimBorder )"
equation "d924 = ( BaseY + Depth + ModuleGap ) + ( ( LeftReach ) - ( ( ( ( ( LeftReach ) - ( 14 * SlotPitch + SlotWidth ) ) / 2 ) + ( 4 * SlotPitch ) ) + ( SlotWidth ) ) )"
equation "d925 = ( LeftSideDepth ) - 2 * ( Wall + DeckClearance + RimBorder )"
equation "d926 = SlotWidth"
equation "d927 = DeckThick"
equation "d929 = ( FootHeight ) + PanHeight - DeckThick"
equation "d931 = ( BaseX ) + ( Wall + DeckClearance + RimBorder )"
equation "d932 = ( BaseY + Depth + ModuleGap ) + ( ( LeftReach ) - ( ( ( ( ( LeftReach ) - ( 14 * SlotPitch + SlotWidth ) ) / 2 ) + ( 5 * SlotPitch ) ) + ( SlotWidth ) ) )"
equation "d933 = ( LeftSideDepth ) - 2 * ( Wall + DeckClearance + RimBorder )"
equation "d934 = SlotWidth"
equation "d935 = DeckThick"
equation "d937 = ( FootHeight ) + PanHeight - DeckThick"
equation "d939 = ( BaseX ) + ( Wall + DeckClearance + RimBorder )"
equation "d940 = ( BaseY + Depth + ModuleGap ) + ( ( LeftReach ) - ( ( ( ( ( LeftReach ) - ( 14 * SlotPitch + SlotWidth ) ) / 2 ) + ( 6 * SlotPitch ) ) + ( SlotWidth ) ) )"
equation "d941 = ( LeftSideDepth ) - 2 * ( Wall + DeckClearance + RimBorder )"
equation "d942 = SlotWidth"
equation "d943 = DeckThick"
equation "d945 = ( FootHeight ) + PanHeight - DeckThick"
equation "d947 = ( BaseX ) + ( Wall + DeckClearance + RimBorder )"
equation "d948 = ( BaseY + Depth + ModuleGap ) + ( ( LeftReach ) - ( ( ( ( ( LeftReach ) - ( 14 * SlotPitch + SlotWidth ) ) / 2 ) + ( 7 * SlotPitch ) ) + ( SlotWidth ) ) )"
equation "d949 = ( LeftSideDepth ) - 2 * ( Wall + DeckClearance + RimBorder )"
equation "d950 = SlotWidth"
equation "d951 = DeckThick"
equation "d953 = ( FootHeight ) + PanHeight - DeckThick"
equation "d955 = ( BaseX ) + ( Wall + DeckClearance + RimBorder )"
equation "d956 = ( BaseY + Depth + ModuleGap ) + ( ( LeftReach ) - ( ( ( ( ( LeftReach ) - ( 14 * SlotPitch + SlotWidth ) ) / 2 ) + ( 8 * SlotPitch ) ) + ( SlotWidth ) ) )"
equation "d957 = ( LeftSideDepth ) - 2 * ( Wall + DeckClearance + RimBorder )"
equation "d958 = SlotWidth"
equation "d959 = DeckThick"
equation "d961 = ( FootHeight ) + PanHeight - DeckThick"
equation "d963 = ( BaseX ) + ( Wall + DeckClearance + RimBorder )"
equation "d964 = ( BaseY + Depth + ModuleGap ) + ( ( LeftReach ) - ( ( ( ( ( LeftReach ) - ( 14 * SlotPitch + SlotWidth ) ) / 2 ) + ( 9 * SlotPitch ) ) + ( SlotWidth ) ) )"
equation "d965 = ( LeftSideDepth ) - 2 * ( Wall + DeckClearance + RimBorder )"
equation "d966 = SlotWidth"
equation "d967 = DeckThick"
equation "d969 = ( FootHeight ) + PanHeight - DeckThick"
equation "d971 = ( BaseX ) + ( Wall + DeckClearance + RimBorder )"
equation "d972 = ( BaseY + Depth + ModuleGap ) + ( ( LeftReach ) - ( ( ( ( ( LeftReach ) - ( 14 * SlotPitch + SlotWidth ) ) / 2 ) + ( 10 * SlotPitch ) ) + ( SlotWidth ) ) )"
equation "d973 = ( LeftSideDepth ) - 2 * ( Wall + DeckClearance + RimBorder )"
equation "d974 = SlotWidth"
equation "d975 = DeckThick"
equation "d977 = ( FootHeight ) + PanHeight - DeckThick"
equation "d979 = ( BaseX ) + ( Wall + DeckClearance + RimBorder )"
equation "d980 = ( BaseY + Depth + ModuleGap ) + ( ( LeftReach ) - ( ( ( ( ( LeftReach ) - ( 14 * SlotPitch + SlotWidth ) ) / 2 ) + ( 11 * SlotPitch ) ) + ( SlotWidth ) ) )"
equation "d981 = ( LeftSideDepth ) - 2 * ( Wall + DeckClearance + RimBorder )"
equation "d982 = SlotWidth"
equation "d983 = DeckThick"
equation "d985 = ( FootHeight ) + PanHeight - DeckThick"
equation "d987 = ( BaseX ) + ( Wall + DeckClearance + RimBorder )"
equation "d988 = ( BaseY + Depth + ModuleGap ) + ( ( LeftReach ) - ( ( ( ( ( LeftReach ) - ( 14 * SlotPitch + SlotWidth ) ) / 2 ) + ( 12 * SlotPitch ) ) + ( SlotWidth ) ) )"
equation "d989 = ( LeftSideDepth ) - 2 * ( Wall + DeckClearance + RimBorder )"
equation "d990 = SlotWidth"
equation "d991 = DeckThick"
equation "d993 = ( FootHeight ) + PanHeight - DeckThick"
equation "d995 = ( BaseX ) + ( Wall + DeckClearance + RimBorder )"
equation "d996 = ( BaseY + Depth + ModuleGap ) + ( ( LeftReach ) - ( ( ( ( ( LeftReach ) - ( 14 * SlotPitch + SlotWidth ) ) / 2 ) + ( 13 * SlotPitch ) ) + ( SlotWidth ) ) )"
equation "d997 = ( LeftSideDepth ) - 2 * ( Wall + DeckClearance + RimBorder )"
equation "d998 = SlotWidth"
equation "d999 = DeckThick"
equation "d1001 = ( FootHeight ) + PanHeight - DeckThick"
equation "d1003 = ( BaseX ) + ( Wall + DeckClearance + RimBorder )"
equation "d1004 = ( BaseY + Depth + ModuleGap ) + ( ( LeftReach ) - ( ( ( ( ( LeftReach ) - ( 14 * SlotPitch + SlotWidth ) ) / 2 ) + ( 14 * SlotPitch ) ) + ( SlotWidth ) ) )"
equation "d1005 = ( LeftSideDepth ) - 2 * ( Wall + DeckClearance + RimBorder )"
equation "d1006 = SlotWidth"
equation "d1007 = DeckThick"
equation "d1009 = ( FootHeight ) + PanHeight - DeckThick"
equation "d1011 = ( BaseX ) + ( ( LeftSideDepth ) - Wall - DeckClearance - 4 mm )"
equation "d1012 = ( BaseY + Depth + ModuleGap ) + ( ( LeftReach ) - ( ( ( LeftReach ) / 2 - 8 mm ) + ( 16 mm ) ) )"
equation "d1015 = DeckThick"
equation "d1017 = TouchChamfer"
equation "d1018 = FootHeight"
equation "d1020 = ( BaseX + LeftRun + FaucetGap + RightRun - RightSideDepth ) + ( ( RightSideDepth ) - ( ( 0 mm ) + ( RightSideDepth ) ) )"
equation "d1021 = ( BaseY + Depth + ModuleGap ) + ( 0 mm )"
equation "d1022 = RightSideDepth"
equation "d1023 = RightReach"
equation "d1024 = PanHeight"
equation "d1028 = ( BaseY + Depth + ModuleGap ) + ( Wall )"
equation "d1030 = ( ( BaseX + LeftRun + FaucetGap + RightRun - RightSideDepth ) + ( ( RightSideDepth ) - ( Wall ) ) )"
equation "d1031 = -( -( ( FootHeight ) + FloorMin + ( ( RightSideDepth ) - ( Wall ) ) * tan(DrainSlope) ) )"
equation "d1032 = ( ( BaseX + LeftRun + FaucetGap + RightRun - RightSideDepth ) + ( ( RightSideDepth ) - ( RightSideDepth ) ) )"
equation "d1033 = -( -( ( FootHeight ) + FloorMin + ( ( RightSideDepth ) - ( RightSideDepth ) ) * tan(DrainSlope) ) )"
equation "d1034 = -( -( FootHeight + PanHeight + 1 mm ) )"
equation "d1035 = ( RightReach ) - 2 * Wall"
equation "d1037 = FootHeight"
equation "d1039 = ( BaseX + LeftRun + FaucetGap + RightRun - RightSideDepth ) + ( ( RightSideDepth ) - ( ( Wall ) + ( 12 mm ) ) )"
equation "d1040 = ( BaseY + Depth + ModuleGap ) + ( Wall )"
equation "d1043 = PanHeight - DeckThick"
equation "d1045 = FootHeight"
equation "d1047 = ( BaseX + LeftRun + FaucetGap + RightRun - RightSideDepth ) + ( ( RightSideDepth ) - ( ( ( RightSideDepth ) - Wall - 12 mm ) + ( 12 mm ) ) )"
equation "d1048 = ( BaseY + Depth + ModuleGap ) + ( Wall )"
equation "d1051 = PanHeight - DeckThick"
equation "d1053 = FootHeight"
equation "d1055 = ( BaseX + LeftRun + FaucetGap + RightRun - RightSideDepth ) + ( ( RightSideDepth ) - ( ( Wall ) + ( 12 mm ) ) )"
equation "d1056 = ( BaseY + Depth + ModuleGap ) + ( ( RightReach ) - Wall - 12 mm )"
equation "d1059 = PanHeight - DeckThick"
equation "d1061 = FootHeight"
equation "d1063 = ( BaseX + LeftRun + FaucetGap + RightRun - RightSideDepth ) + ( ( RightSideDepth ) - ( ( ( RightSideDepth ) - Wall - 12 mm ) + ( 12 mm ) ) )"
equation "d1064 = ( BaseY + Depth + ModuleGap ) + ( ( RightReach ) - Wall - 12 mm )"
equation "d1067 = PanHeight - DeckThick"
equation "d1071 = ( BaseX + LeftRun + FaucetGap + RightRun - RightSideDepth ) + ( ( RightSideDepth ) - ( ( 0 mm ) + ( ( RightSideDepth ) - 9 mm ) ) )"
equation "d1072 = ( BaseY + Depth + ModuleGap ) + ( 3 mm )"
equation "d1073 = ( RightSideDepth ) - 9 mm"
equation "d1074 = RunnerWidth"
equation "d1075 = FootHeight"
equation "d1079 = ( BaseX + LeftRun + FaucetGap + RightRun - RightSideDepth ) + ( ( RightSideDepth ) - ( ( 0 mm ) + ( ( RightSideDepth ) - 9 mm ) ) )"
equation "d1080 = ( BaseY + Depth + ModuleGap ) + ( ( RightReach ) - 3 mm - RunnerWidth )"
equation "d1081 = ( RightSideDepth ) - 9 mm"
equation "d1082 = RunnerWidth"
equation "d1083 = FootHeight"
equation "d1085 = TouchChamfer"
equation "d1086 = ( FootHeight ) + PanHeight - DeckThick"
equation "d1088 = ( BaseX + LeftRun + FaucetGap + RightRun - RightSideDepth ) + ( ( RightSideDepth ) - ( ( Wall + DeckClearance ) + ( ( RightSideDepth ) - 2 * ( Wall + DeckClearance ) ) ) )"
equation "d1089 = ( BaseY + Depth + ModuleGap ) + ( Wall + DeckClearance )"
equation "d1090 = ( RightSideDepth ) - 2 * ( Wall + DeckClearance )"
equation "d1091 = ( RightReach ) - 2 * ( Wall + DeckClearance )"
equation "d1092 = DeckThick"
equation "d1094 = ( FootHeight ) + PanHeight - DeckThick"
equation "d1096 = ( BaseX + LeftRun + FaucetGap + RightRun - RightSideDepth ) + ( ( RightSideDepth ) - ( ( Wall + DeckClearance + RimBorder ) + ( ( RightSideDepth ) - 2 * ( Wall + DeckClearance + RimBorder ) ) ) )"
equation "d1097 = ( BaseY + Depth + ModuleGap ) + ( ( ( ( RightReach ) - ( 14 * SlotPitch + SlotWidth ) ) / 2 ) + ( 0 * SlotPitch ) )"
equation "d1098 = ( RightSideDepth ) - 2 * ( Wall + DeckClearance + RimBorder )"
equation "d1099 = SlotWidth"
equation "d1100 = DeckThick"
equation "d1102 = ( FootHeight ) + PanHeight - DeckThick"
equation "d1104 = ( BaseX + LeftRun + FaucetGap + RightRun - RightSideDepth ) + ( ( RightSideDepth ) - ( ( Wall + DeckClearance + RimBorder ) + ( ( RightSideDepth ) - 2 * ( Wall + DeckClearance + RimBorder ) ) ) )"
equation "d1105 = ( BaseY + Depth + ModuleGap ) + ( ( ( ( RightReach ) - ( 14 * SlotPitch + SlotWidth ) ) / 2 ) + ( 1 * SlotPitch ) )"
equation "d1106 = ( RightSideDepth ) - 2 * ( Wall + DeckClearance + RimBorder )"
equation "d1107 = SlotWidth"
equation "d1108 = DeckThick"
equation "d1110 = ( FootHeight ) + PanHeight - DeckThick"
equation "d1112 = ( BaseX + LeftRun + FaucetGap + RightRun - RightSideDepth ) + ( ( RightSideDepth ) - ( ( Wall + DeckClearance + RimBorder ) + ( ( RightSideDepth ) - 2 * ( Wall + DeckClearance + RimBorder ) ) ) )"
equation "d1113 = ( BaseY + Depth + ModuleGap ) + ( ( ( ( RightReach ) - ( 14 * SlotPitch + SlotWidth ) ) / 2 ) + ( 2 * SlotPitch ) )"
equation "d1114 = ( RightSideDepth ) - 2 * ( Wall + DeckClearance + RimBorder )"
equation "d1115 = SlotWidth"
equation "d1116 = DeckThick"
equation "d1118 = ( FootHeight ) + PanHeight - DeckThick"
equation "d1120 = ( BaseX + LeftRun + FaucetGap + RightRun - RightSideDepth ) + ( ( RightSideDepth ) - ( ( Wall + DeckClearance + RimBorder ) + ( ( RightSideDepth ) - 2 * ( Wall + DeckClearance + RimBorder ) ) ) )"
equation "d1121 = ( BaseY + Depth + ModuleGap ) + ( ( ( ( RightReach ) - ( 14 * SlotPitch + SlotWidth ) ) / 2 ) + ( 3 * SlotPitch ) )"
equation "d1122 = ( RightSideDepth ) - 2 * ( Wall + DeckClearance + RimBorder )"
equation "d1123 = SlotWidth"
equation "d1124 = DeckThick"
equation "d1126 = ( FootHeight ) + PanHeight - DeckThick"
equation "d1128 = ( BaseX + LeftRun + FaucetGap + RightRun - RightSideDepth ) + ( ( RightSideDepth ) - ( ( Wall + DeckClearance + RimBorder ) + ( ( RightSideDepth ) - 2 * ( Wall + DeckClearance + RimBorder ) ) ) )"
equation "d1129 = ( BaseY + Depth + ModuleGap ) + ( ( ( ( RightReach ) - ( 14 * SlotPitch + SlotWidth ) ) / 2 ) + ( 4 * SlotPitch ) )"
equation "d1130 = ( RightSideDepth ) - 2 * ( Wall + DeckClearance + RimBorder )"
equation "d1131 = SlotWidth"
equation "d1132 = DeckThick"
equation "d1134 = ( FootHeight ) + PanHeight - DeckThick"
equation "d1136 = ( BaseX + LeftRun + FaucetGap + RightRun - RightSideDepth ) + ( ( RightSideDepth ) - ( ( Wall + DeckClearance + RimBorder ) + ( ( RightSideDepth ) - 2 * ( Wall + DeckClearance + RimBorder ) ) ) )"
equation "d1137 = ( BaseY + Depth + ModuleGap ) + ( ( ( ( RightReach ) - ( 14 * SlotPitch + SlotWidth ) ) / 2 ) + ( 5 * SlotPitch ) )"
equation "d1138 = ( RightSideDepth ) - 2 * ( Wall + DeckClearance + RimBorder )"
equation "d1139 = SlotWidth"
equation "d1140 = DeckThick"
equation "d1142 = ( FootHeight ) + PanHeight - DeckThick"
equation "d1144 = ( BaseX + LeftRun + FaucetGap + RightRun - RightSideDepth ) + ( ( RightSideDepth ) - ( ( Wall + DeckClearance + RimBorder ) + ( ( RightSideDepth ) - 2 * ( Wall + DeckClearance + RimBorder ) ) ) )"
equation "d1145 = ( BaseY + Depth + ModuleGap ) + ( ( ( ( RightReach ) - ( 14 * SlotPitch + SlotWidth ) ) / 2 ) + ( 6 * SlotPitch ) )"
equation "d1146 = ( RightSideDepth ) - 2 * ( Wall + DeckClearance + RimBorder )"
equation "d1147 = SlotWidth"
equation "d1148 = DeckThick"
equation "d1150 = ( FootHeight ) + PanHeight - DeckThick"
equation "d1152 = ( BaseX + LeftRun + FaucetGap + RightRun - RightSideDepth ) + ( ( RightSideDepth ) - ( ( Wall + DeckClearance + RimBorder ) + ( ( RightSideDepth ) - 2 * ( Wall + DeckClearance + RimBorder ) ) ) )"
equation "d1153 = ( BaseY + Depth + ModuleGap ) + ( ( ( ( RightReach ) - ( 14 * SlotPitch + SlotWidth ) ) / 2 ) + ( 7 * SlotPitch ) )"
equation "d1154 = ( RightSideDepth ) - 2 * ( Wall + DeckClearance + RimBorder )"
equation "d1155 = SlotWidth"
equation "d1156 = DeckThick"
equation "d1158 = ( FootHeight ) + PanHeight - DeckThick"
equation "d1160 = ( BaseX + LeftRun + FaucetGap + RightRun - RightSideDepth ) + ( ( RightSideDepth ) - ( ( Wall + DeckClearance + RimBorder ) + ( ( RightSideDepth ) - 2 * ( Wall + DeckClearance + RimBorder ) ) ) )"
equation "d1161 = ( BaseY + Depth + ModuleGap ) + ( ( ( ( RightReach ) - ( 14 * SlotPitch + SlotWidth ) ) / 2 ) + ( 8 * SlotPitch ) )"
equation "d1162 = ( RightSideDepth ) - 2 * ( Wall + DeckClearance + RimBorder )"
equation "d1163 = SlotWidth"
equation "d1164 = DeckThick"
equation "d1166 = ( FootHeight ) + PanHeight - DeckThick"
equation "d1168 = ( BaseX + LeftRun + FaucetGap + RightRun - RightSideDepth ) + ( ( RightSideDepth ) - ( ( Wall + DeckClearance + RimBorder ) + ( ( RightSideDepth ) - 2 * ( Wall + DeckClearance + RimBorder ) ) ) )"
equation "d1169 = ( BaseY + Depth + ModuleGap ) + ( ( ( ( RightReach ) - ( 14 * SlotPitch + SlotWidth ) ) / 2 ) + ( 9 * SlotPitch ) )"
equation "d1170 = ( RightSideDepth ) - 2 * ( Wall + DeckClearance + RimBorder )"
equation "d1171 = SlotWidth"
equation "d1172 = DeckThick"
equation "d1174 = ( FootHeight ) + PanHeight - DeckThick"
equation "d1176 = ( BaseX + LeftRun + FaucetGap + RightRun - RightSideDepth ) + ( ( RightSideDepth ) - ( ( Wall + DeckClearance + RimBorder ) + ( ( RightSideDepth ) - 2 * ( Wall + DeckClearance + RimBorder ) ) ) )"
equation "d1177 = ( BaseY + Depth + ModuleGap ) + ( ( ( ( RightReach ) - ( 14 * SlotPitch + SlotWidth ) ) / 2 ) + ( 10 * SlotPitch ) )"
equation "d1178 = ( RightSideDepth ) - 2 * ( Wall + DeckClearance + RimBorder )"
equation "d1179 = SlotWidth"
equation "d1180 = DeckThick"